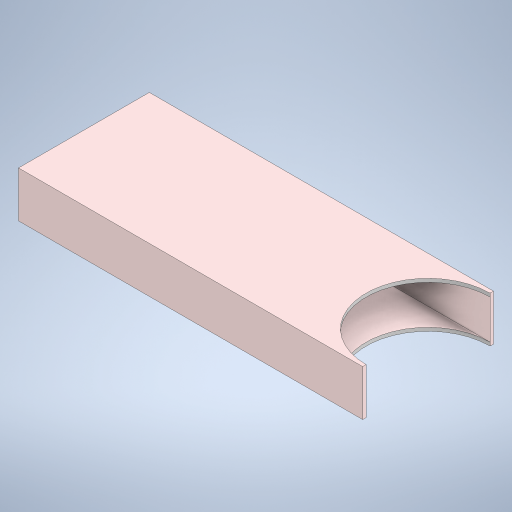
# Autodesk Inventor part: AirIntake
Saved by Autodesk Inventor 2024.3 (Build 283343000, 343)
## iProperties
Created: 2025-03-01
Part Number: AirIntake
Material: Generic
Document SubType Name: Modeling
Designer: ajclo
Density: 1 g/cm^3
Appearance: Default
Author: ajclo
Autodesk Inventor part; units mm, degrees
ref_plane "YZ Plane" through (0, 0, 0) normal (1, 0, 0) x (0, 1, 0)
ref_plane "XZ Plane" through (0, 0, 0) normal (0, 1, 0) x (-1, 0, 0)
ref_plane "XY Plane" through (0, 0, 0) normal (0, 0, 1) x (1, 0, 0)
sketch "Sketch1" plane through (0, 0, 0) normal (1, 0, 0) x (0, 1, 0)
  line L0 (20, 57) -> (-20, 57)
  line L1 (-20, 57) -> (-20, -57)
  line L2 (-20, -57) -> (20, -57)
  line L3 (20, -57) -> (20, 57)
  line L4 (20, 57) -> (-20, -57) construction
  line L5 (-20, 57) -> (20, -57) construction
  line L6 (-17, 54) -> (17, 54)
  line L7 (17, 54) -> (17, -54)
  line L8 (17, -54) -> (-17, -54)
  line L9 (-17, -54) -> (-17, 54)
  line L10 (-17, 54) -> (17, -54) construction
  line L11 (17, 54) -> (-17, -54) construction
  point P0 (0, 0)
  point P1 (0, -57)
  point P2 (0, -54)
  dimension "d0" = 114
  dimension "d1" = 40
  dimension "d2" = 3
  dimension "d3" = 3
  constraints: 24 end point, 6 midpoint, 4 parallel, 2 horizontal, 2 perpendicular
  measures "d0" distance of L2.end L0.start
  measures "d1" distance of L1.end L2.end
  measures "d2" distance between parallel lines of L3 L7
  measures "d3" distance of point (0, -57) point (0, -54)
extrude "Extrusion1" add sketch "Sketch1" along normal blind 300
sketch "Sketch2" plane through (0, 20, 57) normal (0, 1, 0) x (1, 0, 0)
  line L0 (300, 114) -> (300, 0) projected
  circle A0 centre (300, 57) radius 54
  point P0 (0, 57)
  point P1 (300, 111)
  point P2 (300, 3)
  constraints: 1 midpoint, 3 other
extrude "Extrusion2" cut sketch "Sketch2" against normal through all contours L0 A0 picked at (282.6871, 52.0741)
body "Solid1"
